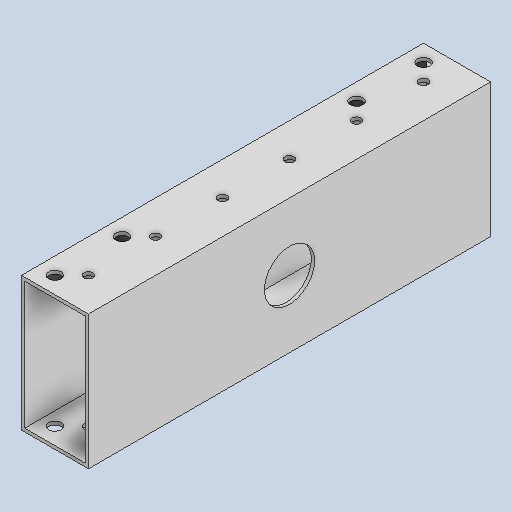
# Autodesk Inventor part: VersaFrame (arm base)
Saved by Autodesk Inventor 2023 (Build 270158000, 158)
## iProperties
Created: 2020-01-13
Part Number: VersaFrame (arm base)
Material: Generic
Document SubType Name: Modeling
Designer: aidan
Density: 1 g/cm^3
Appearance: Default
Mass: 27.4657 g
Surface Area: 440.967 cm^2
Volume: 27.4657 cm^3
Author: aidan
Autodesk Inventor part; units mm, degrees
ref_plane "YZ Plane" through (0, 0, 0) normal (1, 0, 0) x (0, 1, 0)
ref_plane "XZ Plane" through (0, 0, 0) normal (0, 1, 0) x (-1, 0, 0)
ref_plane "XY Plane" through (0, 0, 0) normal (0, 0, 1) x (1, 0, 0)
sketch "Sketch1" plane through (0, 0, 0) normal (0, 0, 1) x (1, 0, 0)
  line L0 (-12.1708, 16.0073) -> (13.2292, 16.0073)
  line L1 (13.2292, 16.0073) -> (13.2292, -34.7927)
  line L2 (13.2292, -34.7927) -> (-12.1708, -34.7927)
  line L3 (-12.1708, -34.7927) -> (-12.1708, 16.0073)
  line L4 (11.9592, 14.7373) -> (-10.9008, 14.7373)
  line L5 (-10.9008, 14.7373) -> (-10.9008, -33.5227)
  line L6 (-10.9008, -33.5227) -> (11.9592, -33.5227)
  line L7 (11.9592, -33.5227) -> (11.9592, 14.7373)
  point P0 (0, 0)
  dimension "d0" = 25.4
  dimension "d1" = 50.8
  dimension "d2" = 1.27
  constraints: 16 end point, 4 parallel, 2 perpendicular, 1 horizontal, 3 other
  measures "d0" distance of L0.start L0.end
  measures "d1" distance of L0.end L1.end
  measures "d2" distance between parallel lines of L0 L4
extrude "Extrusion1" add sketch "Sketch1" along normal blind 152.4
sketch "Sketch2" plane through (-12.1708, 16.0073, 0) normal (0, 1, 0) x (1, 0, 0)
  circle A0 centre (12.7, -12.7) radius 1.7272
  line L0 (25.4, 0) -> (0, 0) projected
  line L1 (0, 0) -> (0, -152.4) projected
  point P0 (12.1708, 0)
  dimension "d5" = 3.4544
  dimension "d6" = 12.7
  dimension "d7" = 12.7
  constraints: 1 centre point
  measures "d5" diameter of A0
  measures "d6" distance from line of L0 A0.centre
  measures "d7" distance from line of L1 A0.centre
extrude "Extrusion2" cut sketch "Sketch2" against normal through all
pattern_linear "Rectangular Pattern1" count 15 spacing 25.4 along (0, 0, 1) of "Extrusion2"
sketch "Sketch3" plane through (-12.1708, 16.0073, 0) normal (0, 1, 0) x (1, 0, 0)
  circle A0 centre (6.35, -6.35) radius 2.3813
  line L0 (25.4, 0) -> (0, 0) projected
  line L1 (0, 0) -> (0, -152.4) projected
  circle A1 centre (6.35, -146.05) radius 2.3813
  line L2 (25.4, -152.4) -> (0, -152.4) projected
  circle A2 centre (6.35, -120.65) radius 2.3813
  circle A3 centre (6.35, -31.75) radius 2.3813
  point P0 (12.1708, 0)
  dimension "d15" = 6.35
  dimension "d16" = 6.35
  dimension "d17" = 4.7625
  dimension "d18" = 6.35
  dimension "d19" = 6.35
  dimension "d20" = 4.7625
  dimension "d23" = 6.35
  dimension "d24" = 6.35
  dimension "d25" = 25.4
  dimension "d26" = 4.7625
  dimension "d27" = 25.4
  dimension "d28" = 4.7625
  constraints: 4 centre point
  measures "d15" distance from line of L0 A0.centre
  measures "d16" distance from line of L1 A0.centre
  measures "d17" diameter of A0
  measures "d18" distance from line of A1.centre L2
  measures "d19" distance from line of L1 A1.centre
  measures "d20" diameter of A1
  measures "d23" distance from line of L1 A2.centre
  measures "d24" distance from line of L1 A3.centre
  measures "d25" distance of A1.centre A2.centre
  measures "d26" diameter of A2
  measures "d27" distance of A0.centre A3.centre
  measures "d28" diameter of A3
extrude "Extrusion3" cut sketch "Sketch3" against normal through all
sketch "Sketch4" plane through (13.2292, -34.7927, 0) normal (1, 0, 0) x (0, 0, -1)
  circle A0 centre (-76.2, 25.4) radius 9.525
  line L0 (0, 0) -> (-152.4, 0) projected
  line L1 (0, 0) -> (0, 50.8) projected
  point P0 (0, 34.7927)
  point P1 (0, 25.4)
  dimension "d29" = 25.4
  dimension "d30" = 76.2
  dimension "d31" = 19.05
  constraints: 1 centre point, 1 midpoint
  measures "d29" distance from line of L0 A0.centre
  measures "d30" distance of point (0, 25.4) A0.centre
  measures "d31" diameter of A0
extrude "Extrusion4" cut sketch "Sketch4" against normal through all
equation "\"d3\" = d13"
equation "\"d10\" = d14"
equation "\"d13\" = 152.4"
equation "\"d14\" = d13"
body "Solid1"
